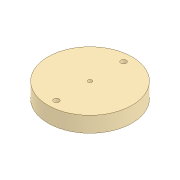
# Autodesk Inventor part: Inferior_encaixe
Saved by Autodesk Inventor 2020 (Build 240168000, 168)
## iProperties
Created: 2022-07-20
Part Number: Inferior_encaixe
Material: Genérico
Document SubType Name: Modeling
Designer: gabri
Density: 1 g/cm^3
Appearance: Bege
Author: gabri
Autodesk Inventor part; units mm, degrees
ref_plane "YZ Plane" through (0, 0, 0) normal (1, 0, 0) x (0, 1, 0)
ref_plane "XZ Plane" through (0, 0, 0) normal (0, 1, 0) x (-1, 0, 0)
ref_plane "XY Plane" through (0, 0, 0) normal (0, 0, 1) x (1, 0, 0)
sketch "Esboço1" plane through (0, 0, 0) normal (0, 1, 0) x (-1, 0, 0)
  circle A0 centre (0, 0) radius 32.5
  circle A1 centre (0, 0) radius 1.5
  dimension "d0" = 65
  dimension "d3" = 3
  constraints: 2 centre point, 2 coincident
  measures "d0" diameter of A0
  measures "d3" diameter of A1
extrude "Extrusão1" add sketch "Esboço1" along normal blind 12
sketch "Esboço2" plane through (0, 0, 0) normal (0, -1, 0) x (1, 0, 0)
  circle A0 centre (0, 0) radius 1.5 projected
  circle A1 centre (0, 0) radius 26
  circle A2 centre (0, -26) radius 2.1
  circle A3 centre (0, 26) radius 2.1
  dimension "d4" = 4.2
  dimension "d5" = 4.2
  dimension "d11" = 52
  constraints: 3 centre point, 2 point on circle, 1 coincident
  measures "d4" diameter of A2
  measures "d5" diameter of A3
  measures "d11" diameter of A1
extrude "Extrusão2" cut sketch "Esboço2" against normal blind 12 contours A3 A1 | A1 A3 | A2 A1 | A1 A2
chamfer "Chanfro1" distance 2.5 angle 45 2 edges at (-2.1, 0, 26) (-2.1, 0, -26)
